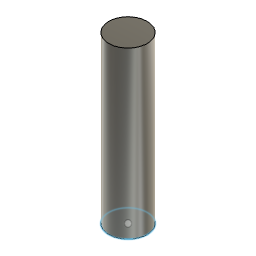
pipette-spring-spacer (Autodesk Fusion 360 design; units mm, degrees)
Autodesk Fusion 360 part; units mm, degrees
sketch "sketch 267" plane through (0, 0, 0) normal (0, 0, 1) x (1, 0, 0)
  circle A0 centre (26.1157, -10.2528) radius 2.9
extrude "Extrude1" add sketch "sketch 267" along normal blind 25
